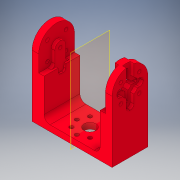
# Autodesk Inventor part: EDMO1-0_Arm
Saved by Autodesk Inventor 2019 (Build 230136000, 136)
## iProperties
Created: 2016-10-25
Part Number: EDMO1-0_Arm
Material: PLA
Document SubType Name: Modeling
Designer: Lucas
Density: 1.29985 g/cm^3
Appearance: Default
Mass: 47.8229 g
Surface Area: 152.012 cm^2
Volume: 36.7911 cm^3
Author: Lucas
Autodesk Inventor part; units mm, degrees
ref_plane "YZ Plane" through (0, 0, 0) normal (1, 0, 0) x (0, 1, 0)
ref_plane "XZ Plane" through (0, 0, 0) normal (0, 1, 0) x (-1, 0, 0)
sketch "Sketch1" plane through (0, 0, 0) normal (0, 0, 1) x (1, 0, 0)
  line L0 (0, 0) -> (47, 0)
  line L1 (47, 0) -> (47, 61.7)
  line L2 (47, 61.7) -> (57, 61.7)
  line L3 (57, 61.7) -> (57, -5)
  line L4 (57, -5) -> (-10, -5)
  line L5 (-10, -5) -> (-10, 61.7)
  line L6 (-10, 61.7) -> (0, 61.7)
  line L7 (0, 61.7) -> (0, 0)
  dimension "d0" = 47
  dimension "d1" = 61.7
  dimension "d2" = 10
  dimension "d13" = 5
  dimension "d64" = 10
  constraints: 16 end point, 5 perpendicular, 2 point on line, 1 horizontal, 1 vertical
  measures "d0" distance of L0.start L0.end
  measures "d1" distance of L0.end L1.end
  measures "d2" distance of L1.end L2.end
  measures "d13" distance between parallel lines of L4 L0
  measures "d64" distance of L5.end L6.end
extrude "Arm_Body" add sketch "Sketch1" along normal blind 30
sketch "Sketch2" plane through (57, -5, 0) normal (1, 0, 0) x (0, 0, -1)
  circle A0 centre (-15, 50.4) radius 1.5
  line L0 (-15, 55.5625) -> (-15, -8.8186) construction
  line L1 (-30, 0) -> (-30, 66.7) projected
  line L2 (0, 66.7) -> (0, 0) projected
  line L3 (0, 66.7) -> (-30, 66.7) projected
  point P0 (0, 5)
  dimension "d7" = 3
  dimension "d8" = 30
  dimension "d9" = 15
  dimension "d10" = 16.3
  constraints: 2 end point, 1 centre point, 1 point on line, 1 vertical
  measures "d7" diameter of A0
  measures "d8" distance between parallel lines of L1 L2
  measures "d9" distance between parallel lines of L0 L2
  measures "d10" distance from line of A0.centre L3
extrude "Shaft_Opening" cut sketch "Sketch2" against normal up to surface (67 mm away)
sketch "Sketch4" plane through (-10, -5, 0) normal (-1, 0, 0) x (0, 0, 1)
  circle A0 centre (15, 50.4) radius 4.5
  circle A1 centre (15, 50.4) radius 1.5 projected
  point P0 (0, 5)
  dimension "d18" = 9
  constraints: 1 centre point, 1 concentric
  measures "d18" diameter of A0
extrude "Pocket_Nut" cut sketch "Sketch4" against normal blind 5.5
sketch "Sketch6" plane through (0, 0, 0) normal (0, 1, 0) x (1, 0, 0)
  circle A0 centre (23.5, -15) radius 11 construction
  line L0 (0, -15) -> (46.0375, -15)
  line L1 (47, -30) -> (0, -30) projected
  line L2 (0, 0) -> (47, 0) projected
  line L3 (0, 0) -> (0, -30) projected
  line L4 (47, 0) -> (47, -30) projected
  circle A1 centre (12.5, -15) radius 1.65
  circle A2 centre (34.5, -15) radius 1.65
  line L5 (9.9716, -1.4716) -> (37.7642, -29.2642) construction
  line L6 (9.808, -28.692) -> (35.7154, -2.7846) construction
  line L7 (23.5, 2.3185) -> (23.5, -31.0285) construction
  circle A3 centre (15.7218, -7.2218) radius 1.65
  circle A4 centre (23.5, -4) radius 1.65
  circle A5 centre (31.2782, -7.2218) radius 1.65
  circle A6 centre (23.5, -26) radius 1.65
  circle A7 centre (15.7218, -22.7782) radius 1.65
  circle A8 centre (31.2782, -22.7782) radius 1.65
  dimension "d21" = 22
  dimension "d22" = 30
  dimension "d23" = 15
  dimension "d24" = 23.5
  dimension "d25" = 47
  dimension "d26" = 3.3
  dimension "d27" = 3.3
  dimension "d28" = 45
  dimension "d29" = 45
  dimension "d30" = 90
  dimension "d31" = 3.3
  dimension "d32" = 3.3
  dimension "d33" = 3.3
  dimension "d34" = 3.3
  dimension "d35" = 3.3
  dimension "d36" = 3.3
  constraints: 12 point on line, 8 centre point, 8 end point, 1 horizontal, 10 other
  measures "d22" distance between parallel lines of L1 L2
  measures "d23" distance between parallel lines of L2 L0
  measures "d24" distance from line of point (23.5, -15) L3
  measures "d25" distance between parallel lines of L4 L3
  measures "d26" diameter of A1
  measures "d27" diameter of A2
  measures "d28" angle of L5 L0
  measures "d29" angle of L0 L6
  measures "d30" angle of L0 L7
  measures "d31" diameter of A3
  measures "d32" diameter of A4
  measures "d33" diameter of A5
  measures "d34" diameter of A6
  measures "d35" diameter of A7
  measures "d36" diameter of A8
extrude "Connector_Holes_Front" cut sketch "Sketch6" against normal up to surface (5 mm away) contours A1 L0 | L0 A1 | A2 L0 | L0 A2 | A3 | A4 | A5 | A6 | A7 | A8
sketch "Sketch8" plane through (47, 0, 4) normal (-1, 0, 0) x (0, 0, 1)
  line L0 (19.4554, 45.6) -> (2.5446, 45.6) construction
  line L1 (11, 58.3863) -> (11, 17.922) construction
  line L2 (14.5, 35.6) -> (14, 27.6)
  line L3 (7.5, 35.6) -> (8, 27.6)
  line L4 (19.4554, 45.6) -> (13.9554, 45.6) construction
  line L5 (2.5446, 45.6) -> (8.0446, 45.6) construction
  line L6 (13, 58.6) -> (9, 58.6) construction
  line L7 (13.9554, 45.6) -> (12.7795, 61.6) construction
  line L8 (8.0446, 45.6) -> (9.2205, 61.6) construction
  line L9 (12.7795, 61.6) -> (9.2205, 61.6) construction
  line L10 (14, 27.6) -> (8, 27.6)
  line L11 (7.5, 35.6) -> (-4, 35.6)
  line L12 (14.5, 35.6) -> (26, 35.6)
  line L13 (-4, 0) -> (-4, 61.7) projected
  line L14 (-4, 35.6) -> (-4, 61.7)
  line L15 (-4, 61.7) -> (26, 61.7) projected
  line L16 (-4, 61.7) -> (26, 61.7)
  line L17 (26, 61.7) -> (26, 35.6)
  point P0 (11, 45.6)
  dimension "d52" = 8
  dimension "d54" = 5.5
  dimension "d55" = 5.5
  dimension "d56" = 4
  dimension "d57" = 13
  dimension "d58" = 16
  dimension "d59" = 16
  dimension "d183" = 10
  dimension "d221" = 10
  dimension "d256" = 15
  dimension "d257" = 3.5
  dimension "d296" = 6
  constraints: 32 end point, 5 point on line, 4 horizontal, 2 collinear, 1 midpoint, 1 parallel, 1 perpendicular, 1 symmetric about line, 1 vertical, 1 other
  measures "d52" vertical distance of L2.start L2.end
  measures "d54" distance of L0.start L4.end
  measures "d55" distance of L0.end L5.end
  measures "d56" distance of L6.start L6.end
  measures "d57" distance between parallel lines of L0 L6
  measures "d58" vertical distance of L4.end L7.end
  measures "d59" vertical distance of L5.end L8.end
  measures "d183" distance between parallel lines of L12 L0
  measures "d221" distance from line of L11 point (11, 45.6)
  measures "d256" distance between parallel lines of L14 L1
  measures "d257" distance from line of L3.start L1
  measures "d296" distance of L2.end L3.end
extrude "Servo_Horn_Pocket" cut sketch "Sketch8" against normal blind 1.5
fillet "Fillet4" radius 2 2 edges at (47.75, 27.6, 12) (47.75, 27.6, 18)
fillet "Fillet9" radius 15 4 edges at (-5, 61.7, 0) (-5, 61.7, 30) (52.75, 61.7, 0) (52.75, 61.7, 30)
sketch "Sketch11" plane through (-10, -5, 0) normal (-1, 0, 0) x (0, 0, 1)
  circle A0 centre (15, 50.4) radius 11 construction
  circle A1 centre (15, 50.4) radius 1.5 projected
  line L0 (1.3636, 36.7636) -> (45.6005, 81.0005) construction
  line L1 (1.3398, 64.0602) -> (31.9798, 33.4202) construction
  line L2 (15, 20.2128) -> (15, 77.3107)
  circle A2 centre (7.2218, 42.6218) radius 1.5
  circle A3 centre (7.2218, 58.1782) radius 1.5
  circle A4 centre (22.7782, 42.6218) radius 1.5
  circle A5 centre (22.7782, 58.1782) radius 1.5
  point P0 (0, 5)
  dimension "d98" = 22
  dimension "d99" = 45
  dimension "d100" = 45
  dimension "d101" = 3
  dimension "d102" = 3
  dimension "d103" = 3
  dimension "d104" = 3
  constraints: 7 point on line, 6 end point, 5 centre point, 4 point on circle, 1 concentric, 1 vertical
  measures "d98" diameter of A0
  measures "d99" angle of L2 L0
  measures "d100" angle of L2 L1
  measures "d101" diameter of A2
  measures "d102" diameter of A3
  measures "d103" diameter of A4
  measures "d104" diameter of A5
extrude "Connector_Holes_Sides" cut sketch "Sketch11" against normal up to surface (67 mm away) contours A2 | A3 | A4 | A5
ref_plane "Work Plane6" through (23.5, 0, 30) normal (1, 0, 0) x (0, 0, -1)
mirror "Mirror7" about plane through (23.5, 0, 30) normal (1, 0, 0) of "Servo_Horn_Pocket", "Fillet4"
sketch "Sketch12" plane through (-10, -5, 0) normal (0, -1, 0) x (1, 0, 0)
  circle A0 centre (33.5, 15) radius 5
  line L0 (0, 0) -> (0, 30) projected
  line L1 (67, 0) -> (67, 30) projected
  line L2 (67, 0) -> (0, 0) projected
  line L3 (0, 30) -> (67, 30) projected
  point P0 (10, 0)
  dimension "d113" = 10
  dimension "d114" = 67
  dimension "d115" = 33.5
  dimension "d116" = 30
  dimension "d117" = 15
  constraints: 1 centre point
  measures "d113" diameter of A0
  measures "d114" distance between parallel lines of L0 L1
  measures "d115" distance from line of A0.centre L1
  measures "d116" distance between parallel lines of L2 L3
  measures "d117" distance from line of L3 A0.centre
extrude "Center_Opening_Front" cut sketch "Sketch12" against normal up to surface (5 mm away) contours A0
fillet "Fillet11" radius 5 2 edges at (47, 0, 15) (0, 0, 15)
sketch "Sketch15" plane through (47, 35.6, 18.5) normal (-1, 0, 0) x (0, 0, 1)
  line L0 (-18.5, -30.6) -> (-18.5, 0) projected
  line L1 (11.5, -40.6) -> (11.5, 11.1) projected
  line L2 (11.5, 11.1) -> (11.5, -30.6) projected
  line L3 (11.5, 5.9218) -> (0.5, 5.9218)
  line L4 (0.5, 5.9218) -> (0.5, -4.0782)
  line L5 (0.5, -4.0782) -> (11.5, -4.0782)
  line L6 (11.5, -4.0782) -> (11.5, 5.9218)
  line L7 (-18.5, 5.9218) -> (-7.5, 5.9218)
  line L8 (-7.5, 5.9218) -> (-7.5, -4.0782)
  line L9 (-7.5, -4.0782) -> (-18.5, -4.0782)
  line L10 (-18.5, -4.0782) -> (-18.5, 5.9218)
  circle A0 centre (-11.2782, 2.0218) radius 1.5 projected
  circle A1 centre (4.2782, 2.0218) radius 1.5 projected
  line L11 (0, 0) -> (-0.3828, -6.1248) projected
  line L12 (-6.6172, -6.1248) -> (-7, 0) projected
  point P0 (-18.5, -35.6)
  point P1 (11.5, 0)
  dimension "d199" = 10
  dimension "d201" = 10
  dimension "d328" = 11
  dimension "d329" = 11
  dimension "d330" = 6.1
  constraints: 16 end point, 4 parallel, 2 horizontal, 2 perpendicular, 2 point on line, 1 collinear
  measures "d199" distance between parallel lines of L5 L3
  measures "d201" distance of L9.end L7.start
  measures "d328" distance of L7.start L7.end
  measures "d329" distance of L3.start L3.end
  measures "d330" distance from line of A0.centre L9
extrude "Nut_Pockets_Sides01" cut sketch "Sketch15" against normal blind 4.5 contours L0 L10 L7 L8 L9 | L5 L4 L3 L1 | A0 | A1
sketch "Sketch16" plane through (48.5, 0, 4) normal (-1, 0, 0) x (0, 0, 1)
  circle A0 centre (18.7782, 53.1782) radius 1.5 projected
  circle A1 centre (3.2218, 53.1782) radius 1.5 projected
  arc A2 (26, 46.7) -> (-4, 46.7) centre (11, 46.7) ccw projected
  line L0 (26, 61.1568) -> (15, 61.1568)
  line L1 (15, 61.1568) -> (15, 50.1782)
  line L2 (15, 50.1782) -> (26, 50.1782)
  line L3 (26, 50.1782) -> (26, 61.1568)
  line L4 (26, 46.7) -> (26, 35.6) projected
  line L5 (7, 61.1568) -> (-4, 61.1568)
  line L6 (-4, 61.1568) -> (-4, 50.1782)
  line L7 (-4, 50.1782) -> (7, 50.1782)
  line L8 (7, 50.1782) -> (7, 61.1568)
  line L9 (-4, 35.6) -> (-4, 46.7) projected
  line L10 (15, 35.6) -> (15, 41.5218) projected
  line L11 (7, 41.5218) -> (7, 35.6) projected
  point P0 (-4, 0)
  point P1 (14, 30.4218)
  dimension "d210" = 3
  dimension "d211" = 3
  constraints: 16 end point, 4 parallel, 3 collinear, 2 horizontal, 2 perpendicular, 2 point on circle, 1 vertical, 1 other
  measures "d210" distance from line of L2 A0.centre
  measures "d211" distance from line of L7 A1.centre
extrude "Nut_Pockets_Sides02" cut sketch "Sketch16" against normal blind 3
sketch "Sketch23" plane through (47, 35.6, 18.5) normal (-1, 0, 0) x (0, 0, 1)
  line L0 (-18.5, -2.7782) -> (11.5, -2.7782)
  line L1 (11.5, -2.7782) -> (11.5, 0)
  line L2 (11.5, 0) -> (-18.5, 0)
  line L3 (-18.5, 0) -> (-18.5, -2.7782)
  line L4 (11.5, 0) -> (0, 0) projected
  line L5 (11.5, 0) -> (11.5, -30.6) projected
  line L6 (-18.5, -30.6) -> (-18.5, 0) projected
  line L7 (-7.5, -4.0782) -> (-18.5, -4.0782) projected
  point P0 (-18.5, -35.6)
  point P1 (11.5, -1.2782)
  dimension "d346" = 1.3
  constraints: 8 end point, 3 collinear, 2 parallel, 1 horizontal, 1 perpendicular
  measures "d346" distance between parallel lines of L0 L7
extrude "Material_Reduction_01" cut sketch "Sketch23" against normal up to surface (1.5 mm away)
sketch "Sketch24" plane through (57, -5, 30) normal (1, 0, 0) x (0, 0, -1)
  circle A0 centre (15, 50.4) radius 4
  line L0 (15, -22.1692) -> (15, 79.8112) construction
  line L1 (30, 51.7) -> (30, 0) projected
  line L2 (0, 0) -> (0, 51.7) projected
  circle A1 centre (15, 50.4) radius 1.5 projected
  point P0 (30, 5)
  dimension "d242" = 8
  dimension "d243" = 30
  dimension "d244" = 15
  dimension "d345" = 0
  constraints: 2 end point, 1 centre point, 1 point on line, 1 vertical
  measures "d242" diameter of A0
  measures "d243" distance between parallel lines of L1 L2
  measures "d244" distance between parallel lines of L0 L2
  measures "d345" distance of A1.centre A0.centre
extrude "Servo_Horn_Opening" cut sketch "Sketch24" against normal up to surface (10 mm away)
mirror "Mirror13" about plane through (23.5, 0, 30) normal (1, 0, 0) of "Material_Reduction_01"
sketch "Sketch25" plane through (48.5, 0, 4) normal (-1, 0, 0) x (0, 0, 1)
  line L0 (15, 41.5218) -> (26, 41.5218) projected
  line L1 (21, 41.5218) -> (26, 41.5218)
  line L2 (26, 41.5218) -> (26, 50.1782)
  line L3 (26, 50.1782) -> (21, 50.1782)
  line L4 (21, 50.1782) -> (21, 41.5218)
  line L5 (1, 41.5218) -> (-4, 41.5218)
  line L6 (-4, 41.5218) -> (-4, 50.1782)
  line L7 (-4, 50.1782) -> (1, 50.1782)
  line L8 (1, 50.1782) -> (1, 41.5218)
  line L9 (-4, 41.5218) -> (-4, 46.7) projected
  line L10 (7, 50.1782) -> (-3.5912, 50.1782) projected
  line L11 (25.5912, 50.1782) -> (15, 50.1782) projected
  line L12 (26, 46.7) -> (26, 41.5218) projected
  point P0 (-4, 0)
  dimension "d341" = 5
  dimension "d342" = 5
  constraints: 16 end point, 4 collinear, 4 parallel, 2 horizontal, 2 perpendicular, 2 point on line
  measures "d341" distance between parallel lines of L6 L8
  measures "d342" distance between parallel lines of L2 L4
extrude "Material_Reduction_02" cut sketch "Sketch25" against normal up to surface (3 mm away)
ref_plane "Work Plane8" through (0, 0, 15) normal (0, 0, 1) x (1, 0, 0)
chamfer "Chamfer3" distance 3.5 distance2 3 1 edges at (50, 41.5218, 11) measured on face at (50, 41.0218, 11)
chamfer "Chamfer4" distance 3.5 distance2 3 1 edges at (50, 41.5218, 19) measured on face at (50, 41.5218, 19.5)
fillet "Fillet20" radius 2 8 edges at (50, 38.5218, 19) (50, 41.5218, 22.5) (49.25, 31.5218, 19) (49.25, 31.5218, 11) (50, 38.0218, 11) (50, 41.5218, 8) (50, 50.1782, 11) (50, 50.1782, 19)
sketch "Sketch27" plane through (57, -5, 30) normal (1, 0, 0) x (0, 0, -1)
  line L0 (-11.7392, 50.4) -> (48.9548, 50.4) construction
  circle A0 centre (15, 50.4) radius 4 construction
  circle A1 centre (15, 50.4) radius 4
  line L1 (15, 78.4425) -> (15, 20.4853) construction
  line L2 (6.5, 51.65) -> (23.5, 51.65) construction
  line L3 (23.5, 51.65) -> (23.5, 49.15)
  line L4 (23.5, 49.15) -> (6.5, 49.15) construction
  line L5 (6.5, 49.15) -> (6.5, 51.65)
  line L6 (13.75, 62.9) -> (16.25, 62.9)
  line L7 (16.25, 62.9) -> (16.25, 37.9) construction
  line L8 (16.25, 37.9) -> (13.75, 37.9)
  line L9 (13.75, 37.9) -> (13.75, 62.9) construction
  arc A2 (30, 51.7) -> (0, 51.7) centre (15, 51.7) ccw projected
  line L10 (6.5, 51.65) -> (13.75, 51.65)
  line L11 (6.5, 49.15) -> (13.75, 49.15)
  line L12 (13.75, 51.65) -> (13.75, 62.9)
  line L13 (16.25, 62.9) -> (16.25, 51.65)
  line L14 (16.25, 51.65) -> (23.5, 51.65)
  line L15 (23.5, 49.15) -> (16.25, 49.15)
  line L16 (16.25, 49.15) -> (16.25, 37.9)
  line L17 (13.75, 37.9) -> (13.75, 49.15)
  circle A3 centre (15, 50.4) radius 4 projected
  point P0 (30, 5)
  dimension "d310" = 2.5
  dimension "d311" = 2.5
  dimension "d312" = 25
  dimension "d313" = 17
  dimension "d314" = 8.5
  dimension "d317" = 12.5
  constraints: 36 end point, 10 point on line, 4 parallel, 4 perpendicular, 3 horizontal, 2 vertical, 1 centre point, 1 coincident, 1 collinear, 1 concentric, 2 other
  measures "d310" distance of L2.end L3.end
  measures "d311" distance of L6.start L6.end
  measures "d312" distance between parallel lines of L8 L6
  measures "d313" distance between parallel lines of L3 L5
  measures "d314" distance between parallel lines of L1 L5
  measures "d317" distance between parallel lines of L6 L0
extrude "Servo_Horn_Screws_Opening" cut sketch "Sketch27" against normal up to surface (8.5 mm away) contours A1 L15 L16 L17 L11 L10 L12 L13 L14 | A1 L14 L3 L15 | A1 L12 L6 L13 | L16 L8 L17 A1 | A1 L11 L5 L10
sketch "Sketch28" plane through (57, -5, 30) normal (1, 0, 0) x (0, 0, -1)
  line L0 (4, 47.15) -> (26, 47.15) construction
  line L1 (26, 47.15) -> (26, 53.65)
  line L2 (26, 53.65) -> (4, 53.65) construction
  line L3 (4, 53.65) -> (4, 47.15)
  arc A0 (18.7997, 51.65) -> (16.25, 54.1997) centre (15, 50.4) ccw projected
  line L4 (4, 47.15) -> (26, 53.65) construction
  line L5 (26, 47.15) -> (4, 53.65) construction
  line L6 (11.75, 34.1) -> (18.25, 34.1)
  line L7 (18.25, 34.1) -> (18.25, 66.7) construction
  line L8 (18.25, 66.7) -> (11.75, 66.7)
  line L9 (11.75, 66.7) -> (11.75, 34.1) construction
  line L10 (11.75, 34.1) -> (18.25, 66.7) construction
  line L11 (18.25, 34.1) -> (11.75, 66.7) construction
  arc A1 (30, 51.7) -> (0, 51.7) centre (15, 51.7) ccw projected
  line L12 (4, 53.65) -> (11.75, 53.65)
  line L13 (4, 47.15) -> (11.75, 47.15)
  line L14 (26, 47.15) -> (18.25, 47.15)
  line L15 (26, 53.65) -> (18.25, 53.65)
  line L16 (11.75, 53.65) -> (11.75, 66.7)
  line L17 (18.25, 53.65) -> (18.25, 66.7)
  line L18 (11.75, 34.1) -> (11.75, 47.15)
  line L19 (18.25, 34.1) -> (18.25, 47.15)
  point P0 (30, 5)
  point P1 (15, 50.4)
  dimension "d318" = 22
  dimension "d319" = 6.5
  dimension "d320" = 6.5
  constraints: 40 end point, 8 point on line, 5 midpoint, 5 parallel, 4 perpendicular, 2 horizontal, 1 collinear, 1 tangent
  measures "d318" distance between parallel lines of L1 L3
  measures "d319" distance between parallel lines of L2 L0
  measures "d320" distance of L7.end L8.end
extrude "Servo_Horn_Screws_Pocket" cut sketch "Sketch28" against normal blind 3
sketch "Sketch29" plane through (57, -5, 30) normal (1, 0, 0) x (0, 0, -1)
  circle A0 centre (15, 50.4) radius 7
  arc A1 (18.7997, 51.65) -> (16.25, 54.1997) centre (15, 50.4) ccw projected
  point P0 (30, 5)
  dimension "d323" = 14
  constraints: 1 centre point, 1 concentric
  measures "d323" diameter of A0
extrude "Extrusion28" cut sketch "Sketch29" against normal up to surface (3 mm away)
fillet "Fillet24" radius 3 6 edges at (55.5, 48.65, 26) (55.5, 42.15, 26) (55.5, 29.1, 18.25) (55.5, 29.1, 11.75) (55.5, 42.15, 4) (55.5, 48.65, 4)
fillet "Fillet25" radius 1 8 edges at (51.25, 44.15, 23.5) (51.25, 46.65, 23.5) (51.25, 44.15, 6.5) (51.25, 46.65, 6.5) (51.25, 32.9, 16.25) (51.25, 32.9, 13.75) (51.25, 57.9, 16.25) (51.25, 57.9, 13.75)
sketch "Sketch30" plane through (-1.5, 46.7, 15) normal (1, 0, 0) x (0, 0, -1)
  line L0 (15, -13.8782) -> (3.3264, -13.8782) projected
  line L1 (15, -13.8782) -> (4.5, -13.8782)
  line L2 (4.5, -13.8782) -> (4.5, 14.3091)
  line L3 (4.5, 14.3091) -> (15, 14.3091)
  line L4 (15, 14.3091) -> (15, -13.8782)
  line L5 (-3.3264, -13.8782) -> (-15, -13.8782) projected
  arc A0 (15, 0) -> (-15, 0) centre (0, 0) ccw projected
  line L6 (-15, -13.8782) -> (-4.5, -13.8782)
  line L7 (-4.5, -13.8782) -> (-4.5, 14.3091)
  line L8 (-4.5, 14.3091) -> (-15, 14.3091)
  line L9 (-15, 14.3091) -> (-15, -13.8782)
  point P0 (15, -46.7)
  dimension "d332" = 10.5
  dimension "d333" = 10.5
  constraints: 16 end point, 4 parallel, 2 horizontal, 2 perpendicular, 2 point on circle
  measures "d332" distance of L2.end L3.end
  measures "d333" distance of L7.end L8.end
extrude "Extrusion29" cut sketch "Sketch30" against normal blind 3 contours L0 L2 A0 L4 | L5 L9 A0 L7 | A0 L9 L8
sketch "Sketch31" plane through (-1.5, 27.6, 16.1211) normal (1, 0, 0) x (0, 0, -1)
  line L0 (5.6211, 22.8) -> (-3.3789, 22.8)
  line L1 (-3.3789, 22.8) -> (-3.3789, 34.1)
  line L2 (-3.3789, 34.1) -> (5.6211, 34.1)
  line L3 (5.6211, 34.1) -> (5.6211, 22.8)
  arc A0 (5.6211, 33.4091) -> (-3.3789, 33.4091) centre (1.1211, 19.1) ccw projected
  circle A1 centre (1.1211, 17.8) radius 1.5 projected
  line L4 (5.6211, 5.2218) -> (5.6211, 33.4091) projected
  line L5 (-3.3789, 33.4091) -> (-3.3789, 5.2218) projected
  point P0 (16.1211, -27.6)
  dimension "d336" = 5
  constraints: 8 end point, 2 collinear, 2 parallel, 1 horizontal, 1 perpendicular, 1 tangent
  measures "d336" distance from line of A1.centre L0
extrude "Extrusion30" cut sketch "Sketch31" against normal up to surface (3 mm away) contours L0 L1 A0 L3
fillet "Fillet27" radius 5 2 edges at (-3, 50.4, 19.5) (-3, 50.4, 10.5)
fillet "Fillet28" radius 3 2 edges at (-3, 32.8218, 19.5) (-3, 32.8218, 10.5)
fillet "Fillet30" radius 2 4 edges at (50, 50.1782, 5) (50, 41.5218, 5) (50, 50.1782, 25) (50, 41.5218, 25)
equation "\"d64\" = d2"
equation "\"d9\" = 0.5 * d8"
equation "\"d23\" = 0.5 * d22"
equation "\"d24\" = 0.5 * d25"
body "Solid1"
